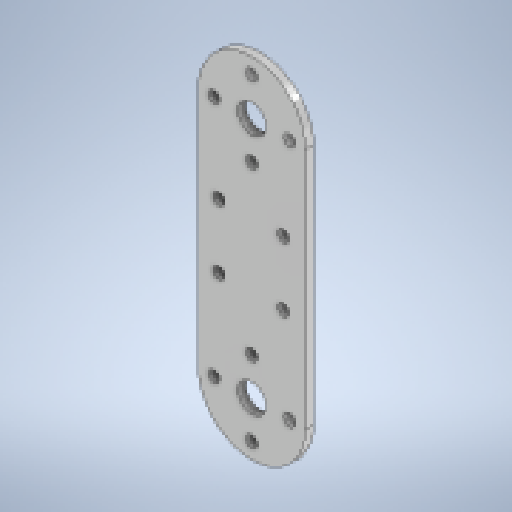
# Autodesk Inventor part: axis_3_bottom_frame(top)
Saved by Autodesk Inventor 2024.1 (Build 281209000, 209)
## iProperties
Created: 2023-09-16
Part Number: axis_3_bottom_frame(top)
Material: Aluminum 6061-AHC
Document SubType Name: Sheet Metal
Designer: chanh
Density: 2.7 g/cm^3
Sheet Metal Rule: Default_mm
Appearance: Aluminum - Dark
Author: chanh
Autodesk Inventor part; units mm, degrees
ref_plane "YZ Plane" through (0, 0, 0) normal (1, 0, 0) x (0, 1, 0)
ref_plane "XZ Plane" through (0, 0, 0) normal (0, 1, 0) x (-1, 0, 0)
ref_plane "XY Plane" through (0, 0, 0) normal (0, 0, 1) x (1, 0, 0)
sketch "Sketch1" plane through (0, 0, 0) normal (0, 0, 1) x (1, 0, 0)
  circle A0 centre (0, 0) radius 9.96
  circle A1 centre (0, 45) radius 9.96
  line L0 (-9.96, 45) -> (-9.96, 0)
  line L1 (9.96, 45) -> (9.96, 0)
  dimension "d0" = 19.92
  dimension "d1" = 45
  measures "d0" diameter of A0
  measures "d1" distance of A1.centre point (0, 0)
extrude "Plate1" add sketch "Sketch1" along normal blind 1.5
sketch "Sketch2" plane through (0, 0, 1.5) normal (0, 0, 1) x (1, 0, 0)
  circle A0 centre (-7, 0) radius 0.7835 projected
  circle A1 centre (7, 0) radius 0.7835 projected
  circle A2 centre (0, 7) radius 0.7835 projected
  circle A3 centre (0, -7) radius 0.7835 projected
  line L0 (-9.96, 0) -> (-9.96, 45) construction
  line L1 (9.96, 45) -> (9.96, 0) construction
  line L2 (-9.96, 22.5) -> (9.96, 22.5) construction
  point P0 (0, 0)
  point P1 (-7, 45)
  point P2 (7, 45)
  point P3 (0, 38)
  point P4 (0, 52)
  constraints: 4 symmetric about line, 2 end point, 2 midpoint
hole "Hole1" at (0, 52, 1.5) at (-7, 45, 1.5) at (0, 38, 1.5) at (7, 45, 1.5) at (0, 7, 1.5) at (-7, 0, 1.5) at (0, -7, 1.5) at (7, 0, 1.5) direction (0, 0, -1) diameter 2.1 end through all
sketch "Sketch3" plane through (0, 0, 1.5) normal (0, 0, 1) x (1, 0, 0)
  circle A0 centre (0, 0) radius 1.75 projected
  circle A1 centre (0, 0) radius 2.6
  line L0 (-9.96, 0) -> (-9.96, 45) construction
  line L1 (9.96, 45) -> (9.96, 0) construction
  line L2 (-9.96, 22.5) -> (9.96, 22.5) construction
  circle A2 centre (0, 45) radius 2.6
  point P0 (0, 0)
  dimension "d10" = 5.2
  constraints: 2 centre point, 2 end point, 2 midpoint, 1 coincident, 1 symmetric about line, 1 other
  measures "d10" diameter of A1
extrude "Extrusion1" cut sketch "Sketch3" against normal through all contours A0 | A1 | A2
sketch "Sketch4" plane through (0, 0, 1.5) normal (0, 0, 1) x (1, 0, 0)
  circle A0 centre (5.865, 29.0135) radius 0.7835 projected
  circle A1 centre (-6.135, 29.0135) radius 0.7835 projected
  circle A2 centre (5.865, 17.1265) radius 0.7835 projected
  circle A3 centre (-6.135, 17.1265) radius 0.7835 projected
  point P0 (0, 0)
hole "Hole2" at (-6.135, 29.0135, 1.5) at (5.865, 29.0135, 1.5) at (-6.135, 17.1265, 1.5) at (5.865, 17.1265, 1.5) direction (0, 0, -1) diameter 2.1 end through all
equation "\"d8\" = Thickness"
equation "\"d18\" = Thickness"
equation "\"d2\" = Thickness"
equation "\"BendReliefWidth\" = Thickness"
equation "\"BendReliefDepth\" = 0.5 * Thickness"
equation "\"CornerReliefSize\" = 4 * Thickness"
equation "\"MinimumRemnant\" = 2 * Thickness"
equation "\"TransitionRadius\" = BendRadius"
equation "\"JacobiRadiusSize\" = BendRadius"
equation "\"GapSize\" = Thickness"
equation "\"Thickness\" = 1.5"
equation "\"BendRadius\" = 0.31"
body "Solid1"
